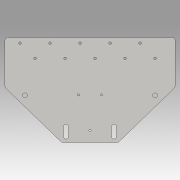
# Autodesk Inventor part: new pulley plate
Saved by Autodesk Inventor 2016 (Build 200138000, 138)
## iProperties
Created: 2015-11-24
Part Number: new pulley plate
Material: Generic
Document SubType Name: Modeling
Designer: Delta
Density: 1 g/cm^3
Appearance: Default
Author: Delta
Autodesk Inventor part; units mm, degrees
ref_plane "YZ Plane" through (0, 0, 0) normal (1, 0, 0) x (0, 1, 0)
ref_plane "XZ Plane" through (0, 0, 0) normal (0, 1, 0) x (-1, 0, 0)
ref_plane "XY Plane" through (0, 0, 0) normal (0, 0, 1) x (1, 0, 0)
sketch "Sketch1" plane through (0, 0, 0) normal (0, 0, 1) x (1, 0, 0)
  line L0 (0, 0) -> (215.9, 0)
  line L1 (215.9, 0) -> (215.9, 152.4)
  line L2 (215.9, 152.4) -> (0, 152.4)
  line L3 (0, 152.4) -> (0, 0)
  dimension "d0" = 215.9
  dimension "d1" = 152.4
  constraints: 8 end point, 2 parallel, 1 horizontal, 1 perpendicular
  measures "d0" distance of L2.end L1.end
  measures "d1" distance of L1.end L0.end
extrude "Extrusion1" add sketch "Sketch1" along normal blind 3.175
sketch "Sketch2" plane through (0, 0, 3.175) normal (0, 0, 1) x (1, 0, 0)
  line L0 (215.9, 152.4) -> (0, 152.4) construction
  line L1 (107.95, 152.4) -> (107.95, 0) construction
  line L2 (0, 0) -> (215.9, 0) projected
  point P0 (25.273, 59.8875)
  point P1 (77.3049, 7.5)
  point P2 (190.627, 59.8875)
  point P3 (138.5951, 7.5)
  dimension "d5" = 30.6451
  dimension "d7" = 82.677
  dimension "d9" = 52.3875
  dimension "d10" = 7.5
  constraints: 2 end point, 2 symmetric about line, 1 midpoint, 1 vertical
  measures "d5" distance from line of L1 point (77.305, 7.5)
  measures "d7" distance from line of L1 point (25.273, 59.887)
  measures "d9" vertical distance of point (25.273, 59.887) point (77.305, 7.5)
  measures "d10" distance from line of L2 point (77.305, 7.5)
hole "Hole1" at (25.273, 59.8875, 3.175) at (77.3049, 7.5, 3.175) at (190.627, 59.8875, 3.175) at (138.5951, 7.5, 3.175) direction (0, 0, -1) diameter 6.35 end through all
sketch "Sketch3" plane through (0, 0, 3.175) normal (0, 0, 1) x (1, 0, 0)
  line L0 (215.9, 152.4) -> (0, 152.4) projected
  line L1 (107.95, 152.4) -> (107.95, 0)
  line L2 (0, 0) -> (215.9, 0) projected
  line L3 (21.4376, 59.8875) -> (76.2, 7.5) construction
  line L4 (0, 152.4) -> (0, 0) projected
  line L5 (0, 130.175) -> (0, 78.2462)
  line L6 (3.175, 133.35) -> (107.95, 133.35)
  line L7 (0, 133.35) -> (0, 125.3708)
  line L8 (194.4624, 59.8875) -> (139.7, 7.5) construction
  line L9 (215.9, 152.4) -> (215.9, 78.2462)
  line L10 (215.9, 133.35) -> (215.9, 76.9596)
  line L11 (212.725, 133.35) -> (107.95, 133.35)
  line L12 (215.9, 130.175) -> (215.9, 125.3708)
  line L13 (75.9713, 0) -> (107.95, 0)
  line L14 (139.9287, 0) -> (107.95, 0)
  line L15 (215.9, 0) -> (215.9, 152.4) projected
  line L16 (107.95, 56.0437) -> (190.627, 56.0437) construction
  line L17 (0, 0) -> (215.9, 0) projected
  line L18 (143.7779, 0) -> (215.9, 69.9366)
  line L19 (72.1221, 0) -> (0, 69.9366)
  line L20 (0, 152.4) -> (0, 0) projected
  line L21 (72.1221, 0) -> (107.95, 0)
  line L22 (3.175, 133.35) -> (0, 133.35)
  line L23 (212.725, 133.35) -> (215.9, 133.35)
  point P0 (74.6275, 0)
  point P1 (0, 76.9596)
  point P2 (77.9849, 0)
  dimension "d20" = 19.05
  dimension "d36" = 135.881
  dimension "d37" = 135.881
  dimension "d41" = 35.8279
  constraints: 36 end point, 21 point on line, 5 collinear, 5 symmetric about line, 2 horizontal, 2 midpoint, 1 perpendicular, 1 vertical
  measures "d20" distance between parallel lines of L6 L0
  measures "d36" angle of L18 L2
  measures "d37" angle of L19 L2
  measures "d41" distance from line of L1 L19.start
sketch "Sketch4" plane through (0, 0, 3.175) normal (0, 0, 1) x (1, 0, 0)
  arc A0 (80.4798, 20.1806) -> (74.13, 20.1806) centre (77.3049, 20.2) ccw
  circle A1 centre (77.3049, 7.5) radius 3.175 projected
  circle A2 centre (77.3049, 7.5) radius 3.175 projected
  line L0 (3.175, 133.35) -> (212.725, 133.35) projected
  line L1 (107.95, 133.35) -> (107.95, 0) construction
  line L2 (0, 0) -> (215.9, 0) projected
  arc A3 (141.77, 20.176) -> (135.4202, 20.176) centre (138.5951, 20.2) ccw
  arc A4 (74.1357, 7.5165) -> (80.474, 7.4806) centre (77.3049, 7.5) ccw
  circle A5 centre (138.5951, 7.5) radius 3.175 projected
  arc A6 (135.4202, 7.5433) -> (141.77, 7.5433) centre (138.5951, 7.5) ccw
  line L3 (141.77, 20.176) -> (141.77, 7.476)
  circle A7 centre (138.5951, 7.5) radius 3.175 projected
  line L4 (141.77, 20.176) -> (154.47, 20.176) construction
  line L5 (135.4202, 20.176) -> (135.4202, 7.476)
  line L6 (135.4202, 20.176) -> (148.1202, 20.176) construction
  line L7 (80.4798, 20.1806) -> (80.4798, 7.4806)
  line L8 (80.4798, 20.1806) -> (93.1798, 20.1806) construction
  line L9 (74.13, 20.1806) -> (74.1358, 7.4806)
  line L10 (74.13, 20.1806) -> (86.83, 20.1806) construction
  line L11 (74.13, 20.1806) -> (80.4798, 20.1806)
  line L12 (74.1358, 7.4806) -> (80.4798, 7.4806)
  line L13 (135.4202, 7.476) -> (141.77, 7.476)
  line L14 (135.4202, 20.176) -> (141.77, 20.176)
  line L15 (107.95, 0) -> (107.95, 152.4)
  line L16 (215.9, 152.4) -> (0, 152.4) projected
  line L17 (138.5951, 7.5) -> (107.95, 7.5)
  line L18 (138.5951, 20.2) -> (107.95, 20.2)
  line L19 (138.5951, 20.2) -> (169.2402, 20.2) construction
  point P0 (75.9713, 0)
  point P1 (139.9287, 0)
  point P2 (136.525, 7.4971)
  dimension "d29" = 6.35
  dimension "d30" = 12.7
  dimension "d44" = 90
  dimension "d45" = 90
  dimension "d46" = 90
  dimension "d48" = 12.7
  dimension "d49" = 12.7
  dimension "d50" = 12.7
  dimension "d117" = 180
  constraints: 34 end point, 9 point on circle, 6 point on line, 5 equal length, 5 horizontal, 4 centre point, 3 midpoint, 2 coincident, 2 parallel, 1 collinear, 1 perpendicular, 1 symmetric about line, 3 other
  measures "d29" diameter of A0
  measures "d30" distance of A1.centre A0.centre
  measures "d44" angle of L3 L4
  measures "d45" angle of L5 L6
  measures "d46" angle of L7 L8
  measures "d48" distance of L9.start L9.end
  measures "d49" distance of L3.start L3.end
  measures "d50" distance of L5.start L5.end
  measures "d117" angle of L18 L19
extrude "Extrusion3" cut sketch "Sketch3" against normal blind 25.4 contours L9 L23 L11 L1 L0 | L1 L6 L22 L4 L0 | L2 L4 L19 | L18 L15 L2
extrude "Extrusion5" cut sketch "Sketch4" against normal blind 25.4 contours L11 A0 | L7 A1 L9 L11 | A1 L12 A4 L9 | L9 A4 L12 A1 | A4 L12 | L14 A3 | L3 A5 L5 L14 | A5 L13 | A5 L13
fillet "Fillet1" radius 3.175 6 edges at (0, 69.9366, 1.5875) (0, 133.35, 1.5875) (215.9, 133.35, 1.5875) (215.9, 69.9366, 1.5875) (143.7779, 0, 1.5875) (72.1221, 0, 1.5875)
sketch "Sketch5" plane through (0, 0, 3.175) normal (0, 0, 1) x (1, 0, 0)
  line L0 (73.4087, 0) -> (142.4913, 0) projected
  line L1 (73.4087, 0) -> (142.4913, 0)
  line L2 (107.95, 0) -> (107.95, 133.35)
  line L3 (212.725, 133.35) -> (3.175, 133.35) projected
  line L4 (107.95, 0) -> (241.3, 0) construction
  line L5 (107.95, 0) -> (107.95, 30.691)
  line L6 (122.6947, 0) -> (122.6947, 60.5028)
  line L7 (122.6947, 0) -> (183.1975, 0) construction
  circle A0 centre (107.95, 15.3455) radius 1.4986
  point P0 (0, 0)
  point P1 (93.2053, 60.5028)
  dimension "d56" = 90
  dimension "d58" = 90
  dimension "d59" = 60.5028
  dimension "d60" = 2.9972
  dimension "d61" = 14.7447
  dimension "d62" = 14.7447
  dimension "d63" = 60.5028
  constraints: 12 end point, 3 midpoint, 2 coincident, 2 horizontal, 2 perpendicular, 2 point on line, 1 centre point, 1 collinear
  measures "d56" angle of L4 L2
  measures "d58" angle of L7 L6
  measures "d59" distance of L6.start L6.end
  measures "d60" diameter of A0
  measures "d61" distance from line of L2 L6.end
  measures "d62" distance from line of point (93.205, 60.503) L2
  measures "d63" distance from line of L0 point (93.205, 60.503)
hole "Hole2" at (107.95, 15.3455, 3.175) at (93.2053, 60.5028, 3.175) at (122.6947, 60.5028, 3.175) at (107.95, 15.3455, 3.175) at (122.6947, 60.5028, 3.175) direction (0, 0, -1) diameter 2.9972 end through all
sketch "Sketch7" plane through (0, 0, 3.175) normal (0, 0, 1) x (1, 0, 0)
  line L0 (212.725, 133.35) -> (3.175, 133.35) projected
  line L1 (0, 130.175) -> (0, 71.2804) projected
  point P0 (0, 0)
  point P1 (19.05, 126.1872)
  point P2 (38.1, 106.807)
  point P3 (57.15, 126.1872)
  point P4 (76.2, 106.807)
  point P5 (95.25, 126.1872)
  point P6 (114.3, 106.807)
  point P7 (133.35, 126.1872)
  point P8 (152.4, 106.807)
  point P9 (171.45, 126.1872)
  point P10 (190.5, 106.807)
  dimension "d83" = 7.1628
  dimension "d84" = 19.05
  dimension "d85" = 7.1628
  dimension "d89" = 26.543
  dimension "d90" = 26.543
  dimension "d94" = 38.1
  dimension "d95" = 57.15
  dimension "d96" = 76.2
  dimension "d97" = 7.1628
  dimension "d98" = 95.25
  dimension "d99" = 26.543
  dimension "d100" = 114.3
  dimension "d102" = 7.1628
  dimension "d103" = 133.35
  dimension "d104" = 26.543
  dimension "d105" = 152.4
  dimension "d106" = 7.1628
  dimension "d107" = 171.45
  dimension "d108" = 26.543
  dimension "d109" = 190.5
  measures "d83" distance from line of L0 point (19.05, 126.187)
  measures "d84" distance from line of L1 point (19.05, 126.187)
  measures "d85" distance from line of L0 point (57.15, 126.187)
  measures "d89" distance from line of L0 point (38.1, 106.807)
  measures "d90" distance from line of L0 point (76.2, 106.807)
  measures "d94" distance from line of L1 point (38.1, 106.807)
  measures "d95" distance from line of L1 point (57.15, 126.187)
  measures "d96" distance from line of L1 point (76.2, 106.807)
  measures "d97" distance from line of L0 point (95.25, 126.187)
  measures "d98" distance from line of L1 point (95.25, 126.187)
  measures "d99" distance from line of L0 point (114.3, 106.807)
  measures "d100" distance from line of L1 point (114.3, 106.807)
  measures "d102" distance from line of L0 point (133.35, 126.187)
  measures "d103" distance from line of L1 point (133.35, 126.187)
  measures "d104" distance from line of L0 point (152.4, 106.807)
  measures "d105" distance from line of L1 point (152.4, 106.807)
  measures "d106" distance from line of L0 point (171.45, 126.187)
  measures "d107" distance from line of L1 point (171.45, 126.187)
  measures "d108" distance from line of L0 point (190.5, 106.807)
  measures "d109" distance from line of L1 point (190.5, 106.807)
hole "Hole4" at (19.05, 126.1872, 3.175) at (38.1, 106.807, 3.175) at (57.15, 126.1872, 3.175) at (76.2, 106.807, 3.175) at (95.25, 126.1872, 3.175) at (114.3, 106.807, 3.175) at (133.35, 126.1872, 3.175) at (152.4, 106.807, 3.175) at (171.45, 126.1872, 3.175) at (190.5, 106.807, 3.175) direction (0, 0, -1) diameter 3.556 end through all
equation "\"d37\" = d36"
equation "\"d48\" = d30"
equation "\"d49\" = d50"
equation "\"d62\" = d61"
equation "\"d63\" = d59"
equation "\"d85\" = d83"
equation "\"d90\" = d89"
equation "\"d97\" = d83"
equation "\"d99\" = d89"
equation "\"d102\" = d83"
equation "\"d104\" = d89"
equation "\"d106\" = d83"
equation "\"d108\" = d89"
body "Solid1"
